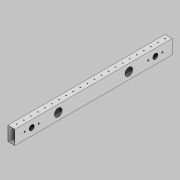
# Autodesk Inventor part: VerseFrame 22.25in for Ball Suck
Saved by Autodesk Inventor 2021 (Build 250183000, 183)
## iProperties
Created: 2020-01-13
Part Number: VerseFrame 22.25in for Ball Suck
Material: Generic
Document SubType Name: Modeling
Designer: aidan
Density: 1 g/cm^3
Appearance: Default
Author: aidan
Autodesk Inventor part; units mm, degrees
ref_plane "YZ Plane" through (0, 0, 0) normal (1, 0, 0) x (0, 1, 0)
ref_plane "XZ Plane" through (0, 0, 0) normal (0, 1, 0) x (-1, 0, 0)
ref_plane "XY Plane" through (0, 0, 0) normal (0, 0, 1) x (1, 0, 0)
sketch "Sketch1" plane through (0, 0, 0) normal (0, 0, 1) x (1, 0, 0)
  line L0 (-12.1708, 16.0073) -> (13.2292, 16.0073)
  line L1 (13.2292, 16.0073) -> (13.2292, -34.7927)
  line L2 (13.2292, -34.7927) -> (-12.1708, -34.7927)
  line L3 (-12.1708, -34.7927) -> (-12.1708, 16.0073)
  line L4 (11.9592, 14.7373) -> (-10.9008, 14.7373)
  line L5 (-10.9008, 14.7373) -> (-10.9008, -33.5227)
  line L6 (-10.9008, -33.5227) -> (11.9592, -33.5227)
  line L7 (11.9592, -33.5227) -> (11.9592, 14.7373)
  point P0 (0, 0)
  dimension "d0" = 25.4
  dimension "d1" = 50.8
  dimension "d2" = 1.27
  constraints: 16 end point, 4 parallel, 2 perpendicular, 1 horizontal, 3 other
  measures "d0" distance of L0.start L0.end
  measures "d1" distance of L0.end L1.end
  measures "d2" distance between parallel lines of L0 L4
extrude "Extrusion1" add sketch "Sketch1" along normal blind 565.15
sketch "Sketch2" plane through (-12.1708, 16.0073, 0) normal (0, 1, 0) x (1, 0, 0)
  circle A0 centre (12.7, -12.7) radius 1.7272
  line L0 (25.4, 0) -> (0, 0) projected
  line L1 (0, 0) -> (0, -565.15) projected
  point P0 (12.1708, 0)
  dimension "d5" = 3.4544
  dimension "d6" = 12.7
  dimension "d7" = 12.7
  constraints: 1 centre point
  measures "d5" diameter of A0
  measures "d6" distance from line of L0 A0.centre
  measures "d7" distance from line of L1 A0.centre
extrude "Extrusion2" cut sketch "Sketch2" against normal through all
pattern_linear "Rectangular Pattern1" count 22 spacing 25.4 along (0, 0, 1) of "Extrusion2"
sketch "Sketch4" plane through (13.2292, -34.7927, 0) normal (1, 0, 0) x (0, 0, -1)
  line L0 (0, 50.8) -> (-565.15, 50.8) construction
  line L1 (-282.575, 50.8) -> (-282.575, 0) construction
  line L2 (0, 0) -> (-565.15, 0) construction
  line L3 (-565.15, 49.53) -> (-565.15, 1.27) construction
  line L4 (-565.15, 25.4) -> (0, 25.4) construction
  line L5 (0, 49.53) -> (0, 1.27) construction
  circle A0 centre (-409.575, 25.4) radius 14.2875
  circle A1 centre (-155.575, 25.4) radius 14.2875
  circle A2 centre (-504.825, 25.4) radius 9.525
  circle A3 centre (-60.325, 25.4) radius 9.525
  circle A4 centre (-530.225, 25.4) radius 2.5781
  circle A5 centre (-479.425, 25.4) radius 2.5781
  circle A6 centre (-85.725, 25.4) radius 2.5781
  circle A7 centre (-34.925, 25.4) radius 2.5781
  point P0 (0, 34.7927)
  dimension "d15" = 28.575
  dimension "d16" = 28.575
  dimension "d17" = 127
  dimension "d18" = 127
  dimension "d19" = 19.05
  dimension "d20" = 19.05
  dimension "d21" = 222.25
  dimension "d22" = 222.25
  dimension "d23" = 5.1562
  dimension "d24" = 5.1562
  dimension "d25" = 25.4
  dimension "d26" = 25.4
  dimension "d27" = 5.1562
  dimension "d28" = 5.1562
  dimension "d29" = 25.4
  dimension "d30" = 25.4
  constraints: 8 centre point, 4 midpoint, 2 end point, 11 other
  measures "d15" diameter of A0
  measures "d16" diameter of A1
  measures "d17" distance from line of L1 A1.centre
  measures "d18" distance from line of L1 A0.centre
  measures "d19" diameter of A2
  measures "d20" diameter of A3
  measures "d21" distance from line of A2.centre L1
  measures "d22" distance from line of L1 A3.centre
  measures "d23" diameter of A4
  measures "d24" diameter of A5
  measures "d25" distance of A2.centre A5.centre
  measures "d26" distance of A4.centre A2.centre
  measures "d27" diameter of A6
  measures "d28" diameter of A7
  measures "d29" distance of A6.centre A3.centre
  measures "d30" distance of A7.centre A3.centre
extrude "Extrusion3" cut sketch "Sketch4" against normal through all
equation "\"d3\" = d13"
equation "\"d10\" = d14"
equation "\"d13\" = 565.15"
equation "\"d14\" = 22.25"
body "Solid1"
